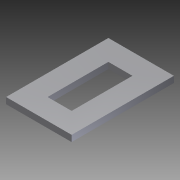
# Autodesk Inventor part: braket servomini
Saved by Autodesk Inventor 2012 (Build 160160000, 160)
## iProperties
Created: 2012-12-01
Part Number: braket servomini
Material: Default
Document SubType Name: Modeling
Designer: irwan
Density: 1 g/cm^3
Author: irwan
Autodesk Inventor part; units mm, degrees
ref_plane "YZ Plane" through (0, 0, 0) normal (1, 0, 0) x (0, 1, 0)
ref_plane "XZ Plane" through (0, 0, 0) normal (0, 1, 0) x (-1, 0, 0)
ref_plane "XY Plane" through (0, 0, 0) normal (0, 0, 1) x (1, 0, 0)
sketch "Sketch1" plane through (0, 0, 0) normal (0, 0, 1) x (1, 0, 0)
  line L0 (0, 0) -> (11.6, 0)
  line L1 (11.6, 0) -> (11.6, 29.3)
  line L2 (11.6, 29.3) -> (0, 29.3)
  line L3 (0, 29.3) -> (0, 0)
  line L4 (-10, 39.3) -> (21.6, 39.3)
  line L5 (21.6, 39.3) -> (21.6, -10)
  line L6 (21.6, -10) -> (-10, -10)
  line L7 (-10, -10) -> (-10, 39.3)
  dimension "d1" = 29.3
  dimension "d5" = 11.6
  dimension "d8" = 10
  constraints: 16 end point, 3 other
  measures "d1" distance of L1.end L0.end
  measures "d5" distance of L0.start L0.end
  measures "d8" distance between parallel lines of L2 L4
extrude "Extrusion1" add sketch "Sketch1" along normal blind 3
body "Solid1"
